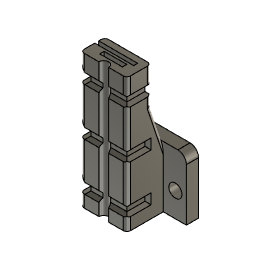
hemera_ribbon_cable_bracket (Autodesk Fusion 360 design; units mm, degrees)
Autodesk Fusion 360 part; units mm, degrees
note: some values were not read from the file. Set by a fixed rule: which face or edge a step refers to.
sketch "Sketch1" plane through (0, 0, 0) normal (0, 0, 1) x (1, 0, 0)
  line L0 (-9.5, -4.95) -> (9.5, -4.95)
  line L1 (9.5, -4.95) -> (9.5, 4.95)
  line L2 (9.5, 4.95) -> (-9.5, 4.95)
  line L3 (-9.5, 4.95) -> (-9.5, -4.95)
  line L4 (-9.5, -4.95) -> (9.5, 4.95) construction
  line L5 (9.5, -4.95) -> (-9.5, 4.95) construction
  line L6 (-9.5, 4.95) -> (-9.5, 2.45)
  line L7 (9.5, 4.95) -> (6.5, 4.95) construction
  line L8 (6.5, 4.95) -> (6.5, -4.95) construction
  line L9 (-9.5, 2.45) -> (6.5, 2.45)
  line L10 (-9.5, 2.45) -> (-9.5, 0.85) construction
  line L11 (-9.5, 0.85) -> (6.5, 0.85)
  line L12 (6.5, 2.45) -> (6.5, 0.85)
  line L13 (-9.5, 0.85) -> (-9.5, -4.95)
  line L14 (-9.5, 0.85) -> (-9.5, -0.15) construction
  line L15 (-9.5, -0.15) -> (9.5, -0.15) construction
  line L16 (0, -0.15) -> (0, -1.05) construction
  line L17 (4.65, -0.1522) -> (-4.65, -0.1522)
  line L18 (-4.65, -0.1522) -> (-4.65, -1.9478)
  line L19 (-4.65, -1.9478) -> (4.65, -1.9478)
  line L20 (4.65, -1.9478) -> (4.65, -0.1522)
  line L21 (4.65, -0.1522) -> (-4.65, -1.9478) construction
  line L22 (-4.65, -0.1522) -> (4.65, -1.9478) construction
  circle A0 centre (0, -4.95) radius 2
  line L23 (6.5, 0.85) -> (6.5, 2.5)
  line L24 (-9.5, 4.95) -> (9.5, 4.95)
  line L25 (9.5, 4.95) -> (9.5, 9.95)
  line L26 (9.5, 9.95) -> (-9.5, 9.95)
  line L27 (-9.5, 9.95) -> (-9.5, 4.95)
  line L28 (0, 9.95) -> (0, 12.45) construction
  line L29 (-19.0023, 9.95) -> (19.0023, 9.95)
  line L30 (19.0023, 9.95) -> (19.0023, 14.95)
  line L31 (19.0023, 14.95) -> (-19.0023, 14.95)
  line L32 (-19.0023, 14.95) -> (-19.0023, 9.95)
  line L33 (-19.0023, 9.95) -> (19.0023, 14.95) construction
  line L34 (19.0023, 9.95) -> (-19.0023, 14.95) construction
  point P0 (0, -1.05)
  point P1 (0, 12.45)
  dimension "d7" = 9.9
  dimension "d8" = 19
  dimension "d9" = 2.5
  dimension "d10" = 3
  dimension "d11" = 1.6
  dimension "d12" = 1
  dimension "d13" = 0.9
  dimension "d14" = 9.3
  dimension "d15" = 4
  dimension "d33" = 5
  dimension "d34" = 2.5
  dimension "d35" = 5
  constraint horizontal L0
  constraint perpendicular L0 L1
  constraint parallel L0 L2
  constraint parallel L1 L3
  constraint coincident L4 origin
  constraint coincident L5 origin
  constraint perpendicular L2 L6
  constraint perpendicular L1 L7
  constraint coincident L0 L8.end
  constraint perpendicular L0 L8
  constraint coincident L8 L9.end
  constraint perpendicular L6 L9
  constraint perpendicular L9 L10
  constraint coincident L8 L11.end
  constraint perpendicular L8 L11
  constraint perpendicular L11 L14
  constraint coincident L1 L15.end
  constraint perpendicular L1 L15
  constraint midpoint L15 L16.start
  constraint perpendicular L15 L16
  constraint horizontal L17
  constraint perpendicular L17 L18
  constraint parallel L17 L19
  constraint parallel L18 L20
  constraint coincident L21 P0
  constraint coincident L22 P0
  constraint coincident P0 L16.end
  constraint midpoint L0 A0.centre
  constraint coincident L8 L23.end
  constraint horizontal L24
  constraint vertical L25
  constraint horizontal L26
  constraint vertical L27
  constraint equal L2 L26
  constraint midpoint L26 L28.start
  constraint perpendicular L26 L28
  constraint horizontal L29
  constraint perpendicular L29 L30
  constraint parallel L29 L31
  constraint parallel L30 L32
  constraint coincident L33 P1
  constraint coincident L34 P1
  constraint coincident P1 L28.end
  measures "d7" distance of L0.end L1.end
  measures "d8" distance of L1.end L2.end
  measures "d9" distance of L2.end L6.end
  measures "d10" distance of L1.end L7.end
  measures "d11" distance of L6.end L10.end
  measures "d12" distance of L10.end L14.end
  measures "d13" distance of L16.start P0
  measures "d14" distance of L18.end L19.end
  measures "d15" diameter of A0
  measures "d33" distance of L2.end L26.end
  measures "d34" distance of L28.start P1
  measures "d35" distance of L29.end L30.end
extrude "Extrude1" add sketch "Sketch1" along normal blind 55 contours L0 L1 L2 L3 L6 L9 L11 L12 L13 A0 L23 L24
extrude "Extrude2" add sketch "Sketch1" along normal blind 2.5 contours L17 L18 L19 L20
ref_plane "WorkPlane1" through (0, 0, 5) normal (0, 0, 1) x (1, 0, 0)
sketch "Sketch2" plane through (0, 0, 5) normal (0, 0, 1) x (1, 0, 0)
  line L0 (-9.5, -4.95) -> (9.5, -4.95)
  line L1 (-9.5, 4.95) -> (-9.5, -4.95)
  line L2 (9.5, 4.95) -> (-9.5, 4.95)
  line L3 (9.5, -4.95) -> (9.5, 4.95)
  line L4 (-9.5, 4.95) -> (-6.5, 4.95)
  line L5 (-6.5, 4.95) -> (-6.5, -4.95) construction
  line L6 (-6.5, -4.95) -> (-9.5, -4.95)
  line L7 (-9.5, -4.95) -> (-9.5, 4.95)
  line L8 (-6.5, 4.95) -> (-6.5, 3.7) construction
  line L9 (-6.5, -4.95) -> (-6.5, -3.7) construction
  line L10 (-6.5, 3.7) -> (9.5, 3.7) construction
  line L11 (-6.5, 4.95) -> (-6.5, -5.4) construction
  line L12 (-6.5, -3.7) -> (9.5, -3.7) construction
  line L13 (9.5, 3.7) -> (8.25, 3.7) construction
  line L14 (8.25, 3.7) -> (8.25, -3.7) construction
  line L15 (8.25, 3.7) -> (-6.5, 3.7)
  line L16 (-6.5, 3.7) -> (-6.5, -3.7)
  line L17 (-6.5, -3.7) -> (8.25, -3.7)
  line L18 (8.25, -3.7) -> (8.25, 3.7)
  line L19 (6.5, 4.95) -> (6.5, -4.95) construction
  dimension "d21" = 3
  dimension "d22" = 1.25
  dimension "d23" = 1.25
  dimension "d24" = 1.25
  constraint horizontal L4
  constraint vertical L5
  constraint horizontal L6
  constraint vertical L7
  constraint coincident L1.start L2.end
  constraint perpendicular L2 L8
  constraint perpendicular L6 L9
  constraint coincident L3 L10.end
  constraint perpendicular L3 L10
  constraint perpendicular L0 L11
  constraint coincident L3 L12.end
  constraint perpendicular L3 L12
  constraint perpendicular L3 L13
  constraint coincident L12 L14.end
  constraint perpendicular L12 L14
  constraint horizontal L15
  constraint vertical L16
  constraint horizontal L17
  constraint vertical L18
  constraint coincident L0.start L6
  measures "d21" distance of L1.start L4.end
  measures "d22" distance of L4.end L8.end
  measures "d23" distance of L5.end L9.end
  measures "d24" distance of L10.end L13.end
extrude "Extrude3" cut sketch "Sketch2" along normal blind 4.25
chamfer "Chamfer1" distance 1.25 angle 45 8 edges at (4.9056, -3.7, 5) (-4.0306, -3.7, 5) (-4.0306, -3.7, 9.25) (4.9056, -3.7, 9.25) (0.875, 3.7, 9.25) (0.875, 3.7, 5) (8.25, 0, 5) (8.25, 0, 9.25)
chamfer "Chamfer2" distance 1.25 angle 45 4 edges at (-6.5, 3.7, 5) (-6.5, -2.05, 5) (-6.5, -2.05, 9.25) (-6.5, 3.7, 9.25)
delete_face "DeleteFace1" 1 faces at (-8.3333, -1.0833, 9.25)
delete_face "DeleteFace2" 1 faces at (-8.3333, 4.1167, 9.25)
pattern_linear "R-Pattern1" count 3 spacing 19.5 along (0, 0, 1) of 20 faces at (-8.9167, 4.1166, 5) (-8.9167, -3.0166, 5) (-7.3334, 3.6999, 5.4166) (-7.3334, 3.6999, 5.4166) (-6.5, 3.2833, 6.8333) (-6.5, -0.6667, 6.8333) (-7.9167, 3.2833, 9.4167) (-5.4168, -4.5333, 8.8336) (-5.4168, -4.5333, 8.8336) (-3.2075, -3.7, 7.4167) (3.7908, -3.7, 6.8333) (-5.4167, -4.5332, 5.4166) (-5.4167, -4.5332, 5.4166) (9.0833, -1.2334, 8.8335) (9.0832, -1.2333, 5.4166) (8.25, 1.2333, 7.4168) (3.3333, 4.5332, 5.4166) (3.3333, 3.7, 6.8333) (3.3333, 4.5332, 8.8334) (-7.9167, 3.2833, 9.4167)
extrude "Extrude4" add sketch "Sketch1" along normal blind 40 contours L2 L24 L25 L26 L27 L29
extrude "Extrude5" add sketch "Sketch1" along normal blind 25 contours L26 L29 L30 L31 L32
hole "Hole1" at (14.5023, 14.95, 10) direction (0, -1, 0) diameter 5.4 end through all
mirror "Mirror1" about plane through (0, 0, 0) normal (1, 0, 0) of "Hole1"
chamfer "Chamfer3" distance 5 distance2 15 1 edges at (0, 9.95, 40) measured on face at (3.1667, 6.6167, 40)
fillet "Fillet1" radius 1.5 10 edges at (-9.5, -4.95, 37.25) (-9.5, -4.95, 52.5) (9.5, -4.95, 51.625) (9.5, 4.95, 51.625) (-9.5, -4.95, 17.75) (-9.5, -4.95, 2.5) (9.5, -4.95, 2.5) (9.5, -4.95, 16.875) (9.5, -4.95, 36.375) (-9.5, 4.95, 52.5)
fillet "Fillet2" radius 1.5 4 edges at (-9.5, 4.95, 42) (-9.5, 7.45, 32.5) (9.5, 4.95, 42) (9.5, 7.45, 32.5)
fillet "Fillet2" radius 1.5 2 edges at (-9.5, 4.95, 27.5) (-9.5, 4.95, 8)
fillet "Fillet2" radius 3.5 2 edges at (-19.0023, 12.45, 25) (19.0023, 12.45, 25)
equation "d7 = 2.5 mm + 1.6 mm + 1 mm + 1.8 mm + 3 mm"
equation "d13 = ( 1.8 / 2 ) * 1 mm"
equation "d36 = 55 mm - 15 mm"
